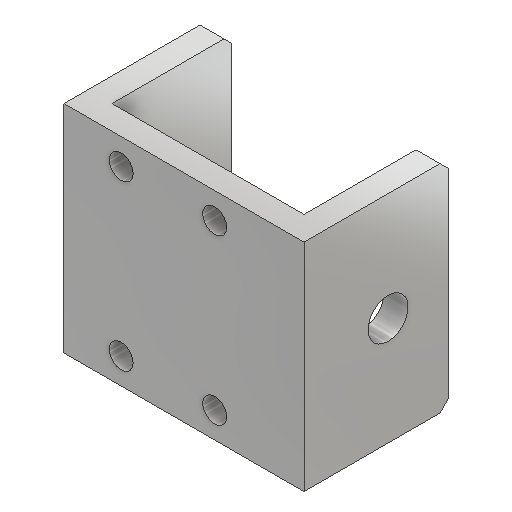
# Autodesk Inventor part: CNCM_ALU_Y_Axis_Tensioning_System_C_Sec
Saved by Autodesk Inventor 2026.1 (Build 301233000, 233)
## iProperties
Created: 2017-08-27
Part Number: CNCM_ALU_Y_Axis_Tensioning_System_C_Sec
Material: Ogólny
Document SubType Name: Modeling
Designer: Andrzej
Density: 1 g/cm^3
Appearance: Aluminium - polerowane
Author: Andrzej
Autodesk Inventor part; units mm, degrees
ref_plane "YZ Plane" through (0, 0, 0) normal (1, 0, 0) x (0, 1, 0)
ref_plane "XZ Plane" through (0, 0, 0) normal (0, 1, 0) x (-1, 0, 0)
ref_plane "XY Plane" through (0, 0, 0) normal (0, 0, 1) x (1, 0, 0)
sketch "Szkic1" plane through (0, 0, 0) normal (0, 0, 1) x (1, 0, 0)
  line L0 (-6.4502, 4.7958) -> (-6.4502, -25.2042)
  line L1 (-6.4502, -25.2042) -> (23.5498, -25.2042)
  line L2 (23.5498, -25.2042) -> (23.5498, 4.7958)
  line L3 (-6.4502, 4.7958) -> (-3.4502, 4.7958)
  line L4 (-3.4502, 4.7958) -> (-3.4502, -22.2042)
  line L5 (23.5498, 4.7958) -> (20.5498, 4.7958)
  line L6 (20.5498, 4.7958) -> (20.5498, -22.2042)
  line L7 (20.5498, -22.2042) -> (-3.4502, -22.2042)
  point P0 (0, 0)
  dimension "d0" = 30
  dimension "d1" = 30
  dimension "d2" = 30
  dimension "d3" = 3
  dimension "d4" = 27
  dimension "d5" = 3
  constraints: 16 end point, 5 perpendicular, 2 horizontal, 1 vertical
  measures "d0" distance of L0.start L0.end
  measures "d1" distance of L0.end L1.end
  measures "d2" distance of L1.end L2.end
  measures "d3" distance of L0.start L3.end
  measures "d4" distance of L3.end L4.end
  measures "d5" distance of L2.end L5.end
extrude "Wyciągnięcie proste1" add sketch "Szkic1" along normal blind 27
sketch "Szkic2" plane through (-6.4502, -25.2042, 0) normal (-1, 0, 0) x (0, 0, 1)
  line L0 (0, 30) -> (0, 0) projected
  line L1 (0, 0) -> (27, 0) projected
  line L2 (27, 30) -> (27, 0) projected
  line L3 (0, 30) -> (27, 30) projected
  line L4 (0, 3) -> (27, 3) projected
  circle A0 centre (13.5, 10.5) radius 2.5
  line L5 (27, 30) -> (27, 0) projected
  line L6 (27, 18) -> (0, 18)
  point P0 (0, 25.2042)
  dimension "d8" = 27
  dimension "d9" = 13.5
  dimension "d10" = 5
  dimension "d11" = 7.5
  dimension "d12" = 7.5
  constraints: 2 end point, 2 point on line, 1 centre point, 1 coincident, 1 perpendicular
  measures "d8" distance of L0.start L2.start
  measures "d9" distance from line of L2 point (13.5, 10.5)
  measures "d10" diameter of A0
  measures "d11" distance from line of L4 A0.centre
  measures "d12" distance from line of point (13.5, 10.5) L6
extrude "Wyciągnięcie proste2" cut sketch "Szkic2" against normal through all contours L3 L2 L6 L0 | A0
chamfer "Faza2" distance 1 angle 45 4 edges at (22.0498, -7.2042, 27) (-4.9502, -7.2042, 27) (22.0498, -7.2042, 0) (-4.9502, -7.2042, 0)
sketch "Szkic5" plane through (-6.4502, -25.2042, 0) normal (0, -1, 0) x (1, 0, 0)
  line L0 (0, 0) -> (30, 0) projected
  line L1 (30, 0) -> (30, 27) projected
  line L2 (0, 27) -> (30, 27) projected
  line L3 (0, 0) -> (0, 27) projected
  line L4 (3, 0) -> (3, 27) projected
  line L5 (27, 0) -> (27, 27) projected
  point P0 (6.4502, 0)
  point P1 (7.15, 23.75)
  point P2 (18.85, 23.75)
  point P3 (7.15, 3.25)
  point P4 (18.85, 3.25)
  dimension "d21" = 20.5
  dimension "d22" = 11.7
  dimension "d24" = 11.7
  dimension "d25" = 20.5
  dimension "d26" = 27
  dimension "d27" = 3.25
  dimension "d28" = 22.85
  constraints: 2 horizontal alignment, 2 vertical alignment
  measures "d21" distance of point (7.15, 3.25) point (7.15, 23.75)
  measures "d22" distance of point (18.85, 23.75) point (7.15, 23.75)
  measures "d24" distance of point (18.85, 3.25) point (7.15, 3.25)
  measures "d25" distance of point (18.85, 3.25) point (18.85, 23.75)
  measures "d26" distance between parallel lines of L0 L2
  measures "d27" distance from line of L2 point (7.15, 23.75)
  measures "d28" distance from line of L1 point (7.15, 23.75)
hole "Otwór1" at (0.6998, -25.2042, 23.75) at (12.3998, -25.2042, 23.75) at (0.6998, -25.2042, 3.25) at (12.3998, -25.2042, 3.25) direction (0, 1, 0) diameter 3 end through all
equation "\"d9\" = 0.5 * d8"
equation "\"d12\" = d11"
equation "\"d27\" = -0.5 * d21 + 0.5 * d26"
